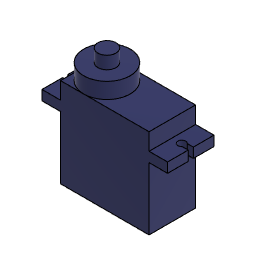
Flap Assy v38 (Autodesk Fusion 360 archive; units mm, degrees)
design "Servo Motor"
Autodesk Fusion 360 part; units mm, degrees
sketch "Sketch1" plane through (0, 0, 0) normal (0, 0, 1) x (1, 0, 0)
  line L0 (11.25, 5.9) -> (-11.25, 5.9)
  line L1 (-11.25, 5.9) -> (-11.25, -5.9)
  line L2 (-11.25, -5.9) -> (11.25, -5.9)
  line L3 (11.25, -5.9) -> (11.25, 5.9)
  line L4 (11.25, 5.9) -> (-11.25, -5.9) construction
  line L5 (-11.25, 5.9) -> (11.25, -5.9) construction
  dimension "d1" = 22.5
  dimension "d2" = 11.8
  constraint horizontal L0
  constraint perpendicular L0 L1
  constraint parallel L0 L2
  constraint parallel L1 L3
  constraint coincident L4 origin
  constraint coincident L5 origin
  measures "d1" distance of L1.end L2.end
  measures "d2" distance of L0.end L1.end
extrude "Extrude1" add sketch "Sketch1" along normal blind 22.7 makes body 1
sketch "Sketch2" plane through (0, 0, 0) normal (0, 0, 1) x (1, 0, 0)
sketch "Sketch3" plane through (0, 0, 0) normal (0, 0, 1) x (1, 0, 0)
  line L0 (-15.95, -5.9) -> (15.95, -5.9)
  line L1 (15.95, -5.9) -> (15.95, 5.9)
  line L2 (15.95, 5.9) -> (-15.95, 5.9)
  line L3 (-15.95, 5.9) -> (-15.95, -5.9)
  line L4 (-15.95, -5.9) -> (15.95, 5.9) construction
  line L5 (15.95, -5.9) -> (-15.95, 5.9) construction
  line L6 (-15.95, 0) -> (-15.95, -0.65) construction
  line L7 (-15.95, -0.65) -> (-13.65, -0.65)
  circle A0 centre (-13.65, 0) radius 1
  line L8 (-15.95, 0) -> (-15.95, 0.65) construction
  line L9 (-15.95, 0.65) -> (-13.65, 0.65)
  line L10 (15.95, 0) -> (15.95, -0.65) construction
  line L11 (15.95, -0.65) -> (13.65, -0.65)
  line L12 (15.95, 0) -> (15.95, 0.65)
  line L13 (15.95, 0.65) -> (13.65, 0.65)
  line L14 (13.65, -0.65) -> (13.65, 0.65) construction
  circle A1 centre (13.65, 0) radius 1
  line L15 (15.95, 0.65) -> (15.95, -0.65)
  line L16 (-15.95, 0.65) -> (-15.95, -0.65)
  dimension "d5" = 31.9
  dimension "d6" = 11.8
  dimension "d9" = 0.65
  dimension "d10" = 2.3
  dimension "d11" = 2
  dimension "d12" = 0.65
  dimension "d13" = 0.65
  dimension "d14" = 2.3
  dimension "d15" = 0.65
  dimension "d16" = 2.3
  dimension "d17" = 2
  constraint horizontal L0
  constraint perpendicular L0 L1
  constraint parallel L0 L2
  constraint parallel L1 L3
  constraint coincident L4 origin
  constraint coincident L5 origin
  constraint midpoint L3 L6.start
  constraint parallel L3 L6
  constraint perpendicular L3 L7
  constraint perpendicular L7 L8
  constraint perpendicular L3 L9
  constraint midpoint L1 L10.start
  constraint parallel L1 L10
  constraint perpendicular L1 L11
  constraint parallel L1 L12
  constraint perpendicular L1 L13
  constraint midpoint L14 A1.centre
  measures "d5" distance of L1.end L2.end
  measures "d6" distance of L0.end L1.end
  measures "d9" distance of L6.start L6.end
  measures "d10" distance of L6.end L7.end
  measures "d11" diameter of A0
  measures "d12" distance of L6.start L8.end
  measures "d13" distance of L10.start L10.end
  measures "d14" distance of L10.end L11.end
  measures "d15" distance of L10.start L12.end
  measures "d16" distance of L12.end L13.end
  measures "d17" diameter of A1
extrude "Extrude2" add sketch "Sketch3" along normal blind 2.5 separate body contours L0 L1 L2 L3 L7 A0 L9 L11 L13 A1 makes body 2
move_body "Move1" bodies 2 to x (1, 0, 0) y (0, 1, 0) z (0, 0, 1) at (0, 0, 15.9)
sketch "Sketch4" plane through (0, 0, 22.7) normal (0, 0, 1) x (-1, 0, 0)
  line L0 (-11.25, 5.9) -> (-11.25, -5.9)
  line L1 (-11.25, -5.9) -> (11.25, -5.9)
  line L2 (11.25, -5.9) -> (11.25, 5.9)
  line L3 (11.25, 5.9) -> (-11.25, 5.9)
  line L4 (11.25, 0) -> (5.35, 0) construction
  circle A0 centre (5.35, 0) radius 5.9
  dimension "d18" = 5.9
  dimension "d19" = 11.8
  constraint midpoint L2 L4.start
  constraint perpendicular L2 L4
  constraint coincident L4.end A0.centre
  measures "d18" distance of L4.start L4.end
  measures "d19" diameter of A0
extrude "Extrude3" add sketch "Sketch4" along normal blind 4 contours A0 bodies 1
combine "Combine1" operation add target body 1 tool bodies 2
sketch "Sketch6" plane through (0, 0, 26.7) normal (0, 0, 1) x (-1, 0, 0)
  circle A0 centre (5.35, 0) radius 5.9
  circle A1 centre (5.35, 0) radius 2.3
  dimension "d22" = 4.6
  constraint concentric A0 A1
  measures "d22" diameter of A1
extrude "Extrude4" add sketch "Sketch6" along normal blind 3.2 contours A1 bodies 1
